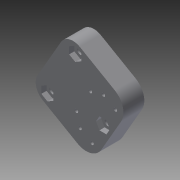
# Autodesk Inventor part: joint3+ax12imprint_v3
Saved by Autodesk Inventor 2014 (Build 180170000, 170)
## iProperties
Created: 2014-01-12
Part Number: joint3+ax12imprint_v3
Material: Générique
Document SubType Name: Modeling
Designer: helly
Density: 1 g/cm^3
Appearance: Par défaut
Author: helly
Autodesk Inventor part; units mm, degrees
ref_plane "YZ Plane" through (0, 0, 0) normal (1, 0, 0) x (0, 1, 0)
ref_plane "XZ Plane" through (0, 0, 0) normal (0, 1, 0) x (-1, 0, 0)
ref_plane "XY Plane" through (0, 0, 0) normal (0, 0, 1) x (1, 0, 0)
sketch "Esquisse1" plane through (0, 0, 0) normal (0, 1, 0) x (-1, 0, 0)
  line L0 (0, 0) -> (32, 0) construction
  line L1 (32, 0) -> (16, 27.7128) construction
  line L2 (16, 27.7128) -> (0, 0) construction
  line L3 (-17.9982, -10.3913) -> (15.6322, 9.0252) construction
  line L4 (11.2583, 6.5) -> (7.2583, 13.4282) construction
  line L5 (11.2583, 6.5) -> (-19.9186, -11.5) construction
  line L6 (-19.9186, -11.5) -> (-26.6686, 0.1913) construction
  line L7 (-26.6686, 0.1913) -> (-21.0394, 3.4413) construction
  line L8 (-21.0394, 3.4413) -> (-14.1112, 7.4413) construction
  line L9 (-14.1112, 7.4413) -> (-7.183, 11.4413) construction
  line L10 (-7.183, 11.4413) -> (-0.2548, 15.4413) construction
  circle A0 centre (-14.1112, 7.4413) radius 1 construction
  circle A1 centre (-7.183, 11.4413) radius 1
  circle A2 centre (-0.2548, 15.4413) radius 1
  circle A3 centre (7.2583, 13.4282) radius 1
  circle A4 centre (-21.0394, 3.4413) radius 1 construction
  circle A5 centre (-0.6112, -15.9413) radius 1 construction
  circle A6 centre (6.317, -11.9413) radius 1
  circle A7 centre (13.2452, -7.9413) radius 1
  circle A8 centre (15.2583, -0.4282) radius 1
  circle A9 centre (-7.5394, -19.9413) radius 1 construction
  circle A10 centre (-19.9186, -11.5) radius 11.6 construction
  line L11 (32, 0) -> (38.9282, 4) construction
  line L12 (36.0415, 0) -> (34.0207, -3.5) construction
  line L13 (34.0207, -3.5) -> (29.9793, -3.5) construction
  line L14 (29.9793, -3.5) -> (27.9585, 0) construction
  line L15 (27.9585, 0) -> (29.9793, 3.5) construction
  line L16 (29.9793, 3.5) -> (34.0207, 3.5) construction
  line L17 (34.0207, 3.5) -> (36.0415, 0) construction
  line L18 (34.0207, 3.5) -> (34.0207, -3.5) construction
  circle A11 centre (16, 27.7128) radius 2
  circle A12 centre (32, 0) radius 2
  line L19 (32, 0) -> (38.9282, 4) construction
  circle A13 centre (0, 0) radius 2
  line L20 (0, 0) -> (11.2583, 6.5) construction
  line L21 (-15.5131, 15.8695) -> (20.1782, 36.476)
  line L22 (20.1782, 36.476) -> (41.6782, -0.7631)
  line L23 (41.6782, -0.7631) -> (5.9869, -21.3695)
  line L24 (-7.183, 11.4413) -> (-11.183, 18.3695) construction
  line L25 (6.317, -11.9413) -> (10.317, -18.8695) construction
  line L26 (6.317, -11.9413) -> (1.9869, -14.4413) construction
  line L27 (-15.5131, 15.8695) -> (5.9869, -21.3695)
  dimension "d0" = 32
  dimension "d1" = 32
  dimension "d2" = 60
  dimension "d4" = 8
  dimension "d6" = 36
  dimension "d7" = 13.5
  dimension "d8" = 6.5
  dimension "d9" = 8
  dimension "d10" = 8
  dimension "d11" = 8
  dimension "d13" = 2
  dimension "d14" = 11.6
  dimension "d15" = 8
  dimension "d16" = 7
  dimension "d17" = 4
  dimension "d19" = 8
  dimension "d69" = 210
  dimension "d70" = 13
  dimension "d83" = 8
  dimension "d84" = 8
  dimension "d85" = 5
  constraints: 57 end point, 14 centre point, 11 coincident, 9 perpendicular, 7 point on line, 6 equal radius, 5 symmetric about line, 4 parallel, 3 collinear, 1 horizontal, 18 other
  measures "d0" distance of L0.start L0.end
  measures "d1" distance of L0.end L1.end
  measures "d2" angle of L1 L0
  measures "d4" distance of L4.start L4.end
  measures "d6" distance of L4.start L5.end
  measures "d7" distance of L5.end L6.end
  measures "d8" distance of L6.end L7.end
  measures "d9" distance of L7.end L8.end
  measures "d10" distance of L8.end L9.end
  measures "d11" distance of L9.end L10.end
  measures "d13" diameter of A4
  measures "d14" radius of A10
  measures "d15" distance of L11.start L11.end
  measures "d16" distance of L16.end L12.end
  measures "d17" diameter of A11
  measures "d19" distance of L19.start L19.end
  measures "d70" distance of L4.start L20.start
  measures "d83" distance of L24.start L24.end
  measures "d84" distance of L25.start L25.end
  measures "d85" distance of L25.start L26.end
extrude "Extrusion7" add sketch "Esquisse1" along normal blind 12
sketch "Esquisse9" plane through (0, 0, 0) normal (0, -1, 0) x (1, 0, 0)
  circle A0 centre (0, 0) radius 2 projected
  circle A1 centre (-32, 0) radius 2 projected
  circle A2 centre (-16, 27.7128) radius 2 projected
  line L0 (-41.6782, -0.7631) -> (-5.9869, -21.3695) projected
  line L1 (18.1112, 14.3695) -> (-3.3888, -22.8695) projected
  line L2 (15.5131, 15.8695) -> (-20.1782, 36.476) projected
  line L3 (-19.5, 25.6921) -> (-19.5, 29.7335)
  line L4 (-19.5, 29.7335) -> (-16, 31.7543)
  line L5 (-16, 31.7543) -> (-12.5, 29.7335)
  line L6 (-12.5, 29.7335) -> (-12.5, 25.6921)
  line L7 (-12.5, 25.6921) -> (-16, 23.6714)
  line L8 (-16, 23.6714) -> (-19.5, 25.6921)
  line L9 (-28.5, 2.0207) -> (-28.5, -2.0207)
  line L10 (-28.5, -2.0207) -> (-32, -4.0415)
  line L11 (-32, -4.0415) -> (-35.5, -2.0207)
  line L12 (-35.5, -2.0207) -> (-35.5, 2.0207)
  line L13 (-35.5, 2.0207) -> (-32, 4.0415)
  line L14 (-32, 4.0415) -> (-28.5, 2.0207)
  line L15 (-19.5, 25.6921) -> (-12.5, 25.6921) construction
  line L16 (4.0415, 0) -> (2.0207, -3.5)
  line L17 (2.0207, -3.5) -> (-2.0207, -3.5)
  line L18 (-2.0207, -3.5) -> (-4.0415, 0)
  line L19 (-4.0415, 0) -> (-2.0207, 3.5)
  line L20 (-2.0207, 3.5) -> (2.0207, 3.5)
  line L21 (2.0207, 3.5) -> (4.0415, 0)
  point P0 (-3.3888, -22.8695)
  dimension "d75" = 7
  constraints: 38 end point, 3 coincident, 3 parallel, 2 equal length, 1 perpendicular, 39 other
  measures "d75" distance of L3.start L6.end
fillet "Congé15" radius 8 1 edges at (-41.6782, 6, -0.7631)
fillet "Congé16" radius 8 1 edges at (-20.1782, 6, 36.476)
extrude "Extrusion8" cut sketch "Esquisse9" against normal blind 3
fillet "Congé17" radius 10 1 edges at (15.5131, 6, 15.8695)
fillet "Congé18" radius 10 1 edges at (-5.9869, 6, -21.3695)
